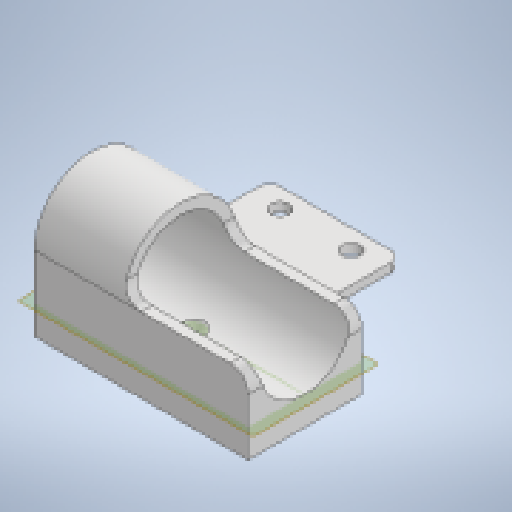
# Autodesk Inventor part: myMotorHolder
Saved by Autodesk Inventor 2023.1 (Build 271208000, 208)
## iProperties
Created: 2025-08-13
Part Number: myMotorHolder
Material: Типовые
Document SubType Name: Modeling
Designer: DELL
Density: 1 g/cm^3
Appearance: По умолчанию
Author: DELL
Autodesk Inventor part; units mm, degrees
ref_plane "YZ Plane" through (0, 0, 0) normal (1, 0, 0) x (0, 1, 0)
ref_plane "XZ Plane" through (0, 0, 0) normal (0, 1, 0) x (-1, 0, 0)
ref_plane "XY Plane" through (0, 0, 0) normal (0, 0, 1) x (1, 0, 0)
sketch "Эскиз1" plane through (0, 0, 0) normal (1, 0, 0) x (0, 1, 0)
  circle A0 centre (0, 0) radius 13
  circle A1 centre (0, 0) radius 16
  line L0 (0, -16) -> (-16, -16)
  line L1 (-16, -16) -> (-16, 16)
  line L2 (-16, 16) -> (0, 16)
  point P0 (-16, 0)
  dimension "d0" = 26
  dimension "d1" = 32
  constraints: 6 end point, 2 centre point, 2 coincident, 2 perpendicular, 2 point on circle, 1 horizontal, 1 tangent
  measures "d0" diameter of A0
  measures "d1" diameter of A1
extrude "Выдавливание1" add sketch "Эскиз1" along normal blind 60 contours A0 | A1 | A1 L1 L2 | L0 L1 A1
sketch "Эскиз2" plane through (60, 0, 0) normal (1, 0, 0) x (0, 0, 1)
  circle A0 centre (0, 0) radius 13
  dimension "d4" = 26
  constraints: 1 centre point, 1 coincident
  measures "d4" diameter of A0
extrude "Выдавливание2" cut sketch "Эскиз2" against normal blind 57
sketch "Эскиз3" plane through (0, 0, 0) normal (-1, 0, 0) x (0, 0, -1)
  circle A0 centre (0, 0) radius 3.6
  circle A1 centre (8.5, 0) radius 1.55
  circle A2 centre (-8.5, 0) radius 1.55
  line L0 (-8.5, 0) -> (8.5, 0) construction
  dimension "d7" = 7.2
  dimension "d8" = 3.1
  dimension "d9" = 3.1
  dimension "d10" = 17
  constraints: 3 centre point, 2 coincident, 2 end point, 1 horizontal, 1 midpoint
  measures "d7" diameter of A0
  measures "d8" diameter of A1
  measures "d9" diameter of A2
  measures "d10" distance of L0.start L0.end
extrude "Выдавливание3" cut sketch "Эскиз3" against normal blind 3
chamfer "Фаска1" distance 1.65 angle 45 2 edges at (0, 0, 10.05) (0, 0, -6.95)
sketch "Эскиз7" plane through (60, 0, 0) normal (1, 0, 0) x (0, 0, -1)
  arc A0 (16, 0) -> (-16, 0) centre (0, 0) ccw projected
  line L0 (-16, 0) -> (16, 0)
  line L1 (16, 0) -> (16, 16)
  line L2 (16, 16) -> (-16, 16)
  line L3 (-16, 16) -> (-16, 0)
  point P0 (16, 0)
  dimension "d25" = 32
  dimension "d26" = 16
  constraints: 8 end point, 2 parallel, 1 horizontal, 1 perpendicular
  measures "d25" distance of L2.end L1.end
  measures "d26" distance of L1.end L0.end
extrude "Выдавливание5" cut sketch "Эскиз7" against normal blind 35 contours L0 A0
fillet "Сопряжение1" radius 5 4 edges at (25, 0, 14.5) (25, 0, -14.5) (60, 0, -14.5) (60, 0, 14.5)
sketch "Эскиз8" plane through (0, -16, -16) normal (0, -1, 0) x (1, 0, 0)
  line L0 (0, 32) -> (60, 32) projected
  line L1 (60, 32) -> (0, 32)
  line L2 (0, 32) -> (0, -34)
  line L3 (0, -34) -> (60, -34)
  line L4 (60, -34) -> (60, 32)
  point P0 (0, 16)
  dimension "d30" = 60
  dimension "d31" = 66
  constraints: 8 end point, 2 parallel, 1 horizontal, 1 perpendicular
  measures "d30" distance of L3.end L2.end
  measures "d31" distance of L2.end L1.end
extrude "Выдавливание6" add sketch "Эскиз8" along normal blind 2.5
sketch "Эскиз9" plane through (0, -18.5, -16) normal (0, -1, 0) x (1, 0, 0)
  line L0 (0, 0) -> (0, 32) projected
  line L1 (0, 0) -> (60, 0)
  line L2 (60, 0) -> (60, 32)
  line L3 (60, 32) -> (0, 32)
  line L4 (0, 32) -> (0, 0)
  point P0 (0, 16)
  constraints: 8 end point, 2 parallel, 1 horizontal, 1 perpendicular
extrude "Выдавливание7" add sketch "Эскиз9" along normal blind 2.5
sketch "Эскиз10" plane through (60, 0, 0) normal (1, 0, 0) x (0, 0, -1)
  line L0 (16, -16) -> (50, -16) projected
  line L1 (16, -18.5) -> (50, -18.5)
  line L2 (50, -18.5) -> (50, -16)
  line L3 (50, -16) -> (16, -16)
  line L4 (16, -16) -> (16, -18.5)
  point P0 (0, 0)
  constraints: 8 end point, 2 parallel, 1 horizontal, 1 perpendicular
extrude "Выдавливание8" cut sketch "Эскиз10" against normal blind 23
sketch "Эскиз11" plane through (0, -16, -16) normal (0, 1, 0) x (1, 0, 0)
  circle A0 centre (28.5, 28.5) radius 2.55
  circle A1 centre (8.5, 28.5) radius 2.55
  circle A2 centre (8.5, 8.5) radius 2.55
  circle A3 centre (28.5, 8.5) radius 2.55
  line L0 (0, 34) -> (37, 34) projected
  line L1 (37, 0) -> (37, 34) projected
  point P0 (0, -16)
  point P1 (3, 34)
  point P2 (34, 34)
  point P3 (37, 3)
  point P4 (37, 31)
  dimension "d39" = 20
  dimension "d41" = 5.1
  dimension "d42" = 5.1
  dimension "d43" = 20
  dimension "d44" = 5.1
  dimension "d45" = 5.1
  dimension "d46" = 20
  dimension "d47" = 5.5
  dimension "d48" = 5.5
  dimension "d49" = 20
  dimension "d51" = 8.5
  dimension "d52" = 8.5
  constraints: 4 centre point
  measures "d39" distance of A0.centre A1.centre
  measures "d41" diameter of A1
  measures "d42" diameter of A0
  measures "d43" distance of A0.centre A3.centre
  measures "d44" diameter of A3
  measures "d45" diameter of A2
  measures "d46" distance of A3.centre A2.centre
  measures "d47" distance from line of L0 A0.centre
  measures "d48" distance from line of L0 A1.centre
  measures "d49" distance of A1.centre A2.centre
  measures "d51" distance from line of L1 A3.centre
  measures "d52" distance from line of L1 A0.centre
extrude "Выдавливание9" cut sketch "Эскиз11" against normal blind 2.5
ref_plane "РабПлоскость2" through (0, -13, -16) normal (0, -1, 0) x (1, 0, 0)
sketch "Эскиз12" plane through (0, -13, -16) normal (0, -1, 0) x (1, 0, 0)
  circle A0 centre (28.5, -8.5) radius 2.55 projected
  line L0 (28.5, -8.5) -> (28.5, 35.2822) construction
  line L1 (60, 32) -> (0, 32) projected
  circle A1 centre (28.5, 16) radius 1.55
  point P0 (0, 16)
  dimension "d56" = 3.1
  dimension "d57" = 16
  constraints: 2 end point, 1 centre point, 1 perpendicular, 1 point on line
  measures "d56" diameter of A1
  measures "d57" distance from line of L1 A1.centre
extrude "Выдавливание10" cut sketch "Эскиз12" along normal mid plane 35 contours A1
chamfer "Фаска2" distance 1.65 angle 45 2 edges at (28.5001, -12.9073, 1.55) (28.3567, -12.9081, -1.5434)
fillet "Сопряжение3" radius 3 4 edges at (18.5, -16, -16) (37, -17.25, -16) (37, -17.25, -50) (0, -17.25, -50)
